Unifi Switch US 8 Mount (Autodesk Fusion 360 design; units mm, degrees)
Autodesk Fusion 360 part; units mm, degrees
note: some values were not read from the file. Set by a fixed rule: which sketch regions a step uses.
sketch "Switch" plane through (0, 0, 0) normal (0, 0, 1) x (1, 0, 0)
  line L0 (0, 0) -> (148, 0)
  line L1 (148, 0) -> (148, 100)
  line L2 (148, 100) -> (0, 100)
  line L3 (0, 100) -> (0, 0)
  line L4 (-3, 100) -> (7, 100)
  line L5 (7, 100) -> (7, -3)
  line L6 (7, -3) -> (-3, -3)
  line L7 (-3, -3) -> (-3, 100)
  line L8 (-3, 100) -> (-18, 100)
  line L9 (-18, 100) -> (-18, 85)
  line L10 (-18, 85) -> (-3, 85)
  line L11 (-3, 85) -> (-3, 100)
  line L12 (-3, -3) -> (-18, -3)
  line L13 (-18, -3) -> (-18, 12)
  line L14 (-18, 12) -> (-3, 12)
  line L15 (-3, 12) -> (-3, -3)
  circle A0 centre (-10.5, 5.75) radius 2
  circle A1 centre (-10.5, 91.25) radius 2
  line L16 (-3, -3) -> (-18, -3)
  line L17 (-18, -3) -> (-18, -0.5)
  line L18 (-18, -0.5) -> (-3, -0.5)
  line L19 (-3, -0.5) -> (-3, -3)
  line L20 (-3, 100) -> (-18, 100)
  line L21 (-18, 100) -> (-18, 97.5)
  line L22 (-18, 97.5) -> (-3, 97.5)
  line L23 (-3, 97.5) -> (-3, 100)
  dimension "d1" = 100
  dimension "d2" = 148
  dimension "d3" = 7
  dimension "d4" = 3
  dimension "d6" = 3
  dimension "d7" = 15
  dimension "d8" = 15
  dimension "d10" = 15
  dimension "d12" = 4
  dimension "d13" = 4
  dimension "d21" = 7.5
  dimension "d31" = 6.25
  dimension "d32" = 15
  dimension "d33" = 2.5
  dimension "d34" = 7.5
  dimension "d35" = 2.5
  dimension "d36" = 6.25
  constraint horizontal L0
  constraint vertical L1
  constraint horizontal L2
  constraint vertical L3
  constraint coincident L0.start L3.end
  constraint horizontal L4
  constraint vertical L5
  constraint horizontal L6
  constraint vertical L7
  constraint horizontal L8
  constraint vertical L9
  constraint vertical L11
  constraint horizontal L12
  constraint vertical L13
  constraint horizontal L14
  constraint vertical L15
  constraint collinear L2 L4
  constraint horizontal L16
  constraint vertical L17
  constraint horizontal L18
  constraint vertical L19
  constraint horizontal L20
  constraint vertical L21
  constraint horizontal L22
  constraint vertical L23
  measures "d1" distance of L0.start L2.end
  measures "d2" distance of L1.end L2.end
  measures "d3" distance of L3 L5
  measures "d4" distance of L3 L7
  measures "d6" distance of L0 L6
  measures "d7" distance of L4.start L8.end
  measures "d8" distance of L8.end L9.end
  measures "d10" distance of L12.end L13.end
  measures "d12" diameter of A0
  measures "d13" diameter of A1
  measures "d21" distance of L7 A1.centre
  measures "d31" distance of L14 A0.centre
  measures "d32" distance of L6.end L12.end
  measures "d33" distance of L6.end L18.end
  measures "d34" distance of L13 A0.centre
  measures "d35" distance of L4.start L22.end
  measures "d36" distance of L10 A1.centre
extrude "Extrude1" add sketch "Switch" along normal blind 33.5 contours L0 L3 L4 L5 L6 L7 L11 L15 L19 L23
extrude "Extrude2" add sketch "Switch" along normal blind 2.5 from surface at 31 contours L0 L2 L3 L4 L5
extrude "Extrude3" add sketch "Switch" along normal blind 2.5 contours L7 L9 L10 L11 L22 | L7 L13 L14 L15 L18
extrude "Extrude5" add sketch "Switch" along normal blind 18 contours L7 L8 L9 L11 L20 L21 L22 L23 | L7 L12 L13 L15 L16 L17 L18 L19
sketch "Venting hole" plane through (0, 0, 0) normal (1, 0, 0) x (0, 1, 0)
  line L0 (92.5, 8.3) -> (6.5, 8.3)
  line L1 (6.5, 8.3) -> (6.5, 21.3)
  line L2 (6.5, 21.3) -> (92.5, 21.3)
  line L3 (92.5, 21.3) -> (92.5, 8.3)
  line L4 (0, 0) -> (0, 31)
  line L5 (100, 0) -> (100, 18)
  point P0 (100, 0)
  dimension "d40" = 8.3
  dimension "d41" = 6.5
  dimension "d42" = 7.5
  dimension "d43" = 13
  constraint horizontal L0
  constraint vertical L1
  constraint horizontal L2
  constraint vertical L3
  measures "d40" distance of L0 P0
  measures "d41" distance of L1 L4
  measures "d42" distance of L3 L5
  measures "d43" distance of L0.end L1.end
extrude "Extrude6" cut sketch "Venting hole" against normal blind 10
fillet "Fillet1" radius 4 4 edges at (-1.5, 6.5, 21.3) (-1.5, 6.5, 8.3) (-1.5, 92.5, 8.3) (-1.5, 92.5, 21.3)
fillet "Fillet2" radius 3 2 edges at (2, -3, 33.5) (2, 100, 33.5)
chamfer "Chamfer1" distance 15 angle 45 2 edges at (-18, 98.75, 18) (-18, -1.75, 18)
fillet "Fillet3" radius 3 2 edges at (-18, 12, 1.25) (-18, 85, 1.25)
